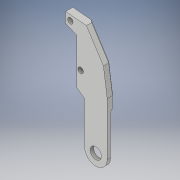
# Autodesk Inventor part: Ladelasche
Saved by Autodesk Inventor 2019 (Build 230136000, 136)
## iProperties
Created: 2021-03-08
Part Number: Ladelasche
Material: Generic
Document SubType Name: Modeling
Designer: Lukas
Density: 1 g/cm^3
Appearance: Default
Author: Lukas
Autodesk Inventor part; units mm, degrees
ref_plane "YZ Plane" through (0, 0, 0) normal (1, 0, 0) x (0, 1, 0)
ref_plane "XZ Plane" through (0, 0, 0) normal (0, 1, 0) x (-1, 0, 0)
ref_plane "XY Plane" through (0, 0, 0) normal (0, 0, 1) x (1, 0, 0)
sketch "Sketch1" plane through (0, 0, 0) normal (0, 0, 1) x (1, 0, 0)
  circle A0 centre (0, -20) radius 6
  circle A1 centre (0, -20) radius 3
  line L0 (-5, 36) -> (4, 22)
  line L1 (-6, -20) -> (-6, 2)
  line L2 (-6, 2) -> (-10, 5)
  line L3 (6, -20) -> (6, 8)
  line L4 (6, 8) -> (4, 22)
  circle A2 centre (-13.5, 34) radius 1.45
  line L5 (-10, 5) -> (-10, 29)
  line L6 (-10, 29) -> (-16, 31.5)
  line L7 (-16, 31.5) -> (-16, 37)
  line L8 (-16, 37) -> (-5, 36)
  point P0 (0, 0)
  point P1 (3.8005, -24.6429)
  dimension "d0" = 6
  dimension "d1" = 12
  dimension "d2" = 20
  dimension "d9" = 3
  dimension "d14" = 22
  dimension "d23" = 2.9
  dimension "d48" = 24
  dimension "d49" = 2.5
  dimension "d50" = 6
  dimension "d55" = 2.5
  dimension "d56" = 3
  dimension "d57" = 8
  dimension "d58" = 22
  dimension "d59" = 36
  dimension "d60" = 4
  dimension "d61" = 10
  dimension "d62" = 5
  dimension "d63" = 37
  constraints: 18 end point, 3 centre point, 3 point on circle, 3 vertical, 2 tangent, 1 coincident, 1 parallel, 1 vertical alignment
  measures "d0" diameter of A1
  measures "d1" diameter of A0
  measures "d2" distance of point (0, 0) A0.centre
  measures "d9" vertical distance of L2.end L1.end
  measures "d14" distance of L1.start L1.end
  measures "d23" diameter of A2
  measures "d48" distance of L2.end L5.end
  measures "d49" vertical distance of L5.end L6.end
  measures "d50" horizontal distance of L5.end L6.end
  measures "d55" distance from line of L7 A2.centre
  measures "d56" vertical distance of L7.end A2.centre
  measures "d57" vertical distance of L3.end point (0, 0)
  measures "d58" vertical distance of L0.end point (0, 0)
  measures "d59" vertical distance of point (0, 0) L0.start
  measures "d60" horizontal distance of L0.end point (0, 0)
  measures "d61" horizontal distance of point (0, 0) L2.end
  measures "d62" horizontal distance of L0.start point (0, 0)
  measures "d63" vertical distance of L7.end point (0, 0)
extrude "Extrusion1" add sketch "Sketch1" along normal blind 1.8
sketch "Sketch2" plane through (0, 0, 1.8) normal (0, 0, 1) x (1, 0, 0)
  line L0 (4, 22) -> (-5, 36) projected
  circle A0 centre (-8, 14) radius 1.45
  line L1 (-10, 29) -> (-10, 5) projected
  point P0 (0, 0)
  dimension "d26" = 9
  dimension "d28" = 2.9
  dimension "d64" = 2
  constraints: 1 centre point
  measures "d26" vertical distance of L1.end A0.centre
  measures "d28" diameter of A0
  measures "d64" distance from line of L1 A0.centre
extrude "Extrusion3" cut sketch "Sketch2" against normal through all
sketch "Sketch3" plane through (0, 0, 0) normal (0, 0, -1) x (-1, 0, 0)
  circle A0 centre (8, 14) radius 1.45 projected
  line L0 (-6, 8) -> (-4, 22) projected
  line L1 (-6, -20) -> (-6, 8) projected
  arc A1 (-6, -20) -> (6, -20) centre (0, -20) ccw projected
  line L2 (6, 2) -> (6, -20) projected
  line L3 (10, 5) -> (6, 2) projected
  line L4 (-4, 22) -> (5, 36) projected
  circle A2 centre (0, -20) radius 3 projected
  circle A3 centre (13.5, 34) radius 1.45 projected
  line L5 (-6, 8) -> (-3.8669, 22.9316) projected
  line L6 (6, -2.5) -> (-6, 1)
  line L7 (6, 2) -> (6, -20) projected
  line L8 (10, 29) -> (10, 5) projected
  line L9 (16, 31.5) -> (10, 29) projected
  line L10 (16, 37) -> (16, 31.5) projected
  line L11 (5, 36) -> (16, 37) projected
  point P0 (0, 0)
  point P1 (-3.6167, 22.8959)
  dimension "d37" = 21
  dimension "d38" = 17.5
  constraints: 2 end point, 2 point on line
  measures "d37" vertical distance of A2.centre L6.end
  measures "d38" vertical distance of L6.start A1.centre
extrude "Extrusion4" add sketch "Sketch3" along normal blind 2 contours L0 L4 L11 L10 L9 L8 L3 L2 L6 L1
chamfer "Chamfer1" distance 2 angle 45 1 edges at (0, -0.75, -2)
chamfer "Chamfer2" distance 1 angle 45 3 edges at (5, 15, -2) (6, 5.5416, -2) (-0.5, 29, -2)
body "Solid1"
